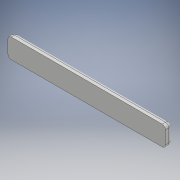
# Autodesk Inventor part: gojung
Saved by Autodesk Inventor 2018 (Build 220112000, 112)
## iProperties
Created: 2019-11-11
Part Number: gojung
Material: 일반
Document SubType Name: Modeling
Designer: LeeYounSeo
Density: 1 g/cm^3
Appearance: 기본값
Author: LeeYounSeo
Autodesk Inventor part; units mm, degrees
ref_plane "YZ Plane" through (0, 0, 0) normal (1, 0, 0) x (0, 1, 0)
ref_plane "XZ Plane" through (0, 0, 0) normal (0, 1, 0) x (-1, 0, 0)
ref_plane "XY Plane" through (0, 0, 0) normal (0, 0, 1) x (1, 0, 0)
sketch "스케치1" plane through (0, 0, 0) normal (0, 1, 0) x (-1, 0, 0)
  line L0 (0, 0) -> (-48, 0)
  line L1 (-48, 0) -> (-48, -6)
  line L2 (-48, -6) -> (0, -6)
  line L3 (0, -6) -> (0, 0)
  dimension "d0" = 48
  dimension "d1" = 6
  constraints: 8 end point, 2 parallel, 1 horizontal, 1 perpendicular
  measures "d0" distance of L1.end L2.end
  measures "d1" distance of L0.end L1.end
extrude "돌출1" add sketch "스케치1" along normal blind 2
fillet "모깎기1" radius 1 7 edges at (0, 1, -6) (0, 1, 0) (0, 2, -3) (24, 2, -6) (48, 2, -3) (24, 2, 0) (48, 1, -6)
fillet "모깎기2" radius 1 2 edges at (47.7071, 1.7071, -0.2929) (48, 0.5, 0)
